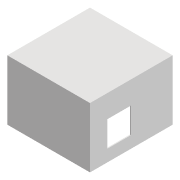
# Autodesk Inventor part: 玻璃罩
Saved by Autodesk Inventor 2021 (Build 250183000, 183)
## iProperties
Created: 2025-04-18
Part Number: 玻璃罩
Material: 常规
Document SubType Name: Modeling
Designer: 86155
Density: 1 g/cm^3
Appearance: 默认
Author: 86155
Autodesk Inventor part; units mm, degrees
ref_plane "YZ Plane" through (0, 0, 0) normal (1, 0, 0) x (0, 1, 0)
ref_plane "XZ Plane" through (0, 0, 0) normal (0, 1, 0) x (-1, 0, 0)
ref_plane "XY Plane" through (0, 0, 0) normal (0, 0, 1) x (1, 0, 0)
sketch "草图1" plane through (0, 0, 0) normal (0, 1, 0) x (-1, 0, 0)
  line L0 (410, 410) -> (-410, 410)
  line L1 (-410, 410) -> (-410, -410)
  line L2 (-410, -410) -> (410, -410)
  line L3 (410, -410) -> (410, 410)
  line L4 (410, 410) -> (-410, -410) construction
  line L5 (-410, 410) -> (410, -410) construction
  line L6 (420, 420) -> (-420, 420)
  line L7 (-420, 420) -> (-420, -420)
  line L8 (-420, -420) -> (420, -420)
  line L9 (420, -420) -> (420, 420)
  point P0 (0, 0)
  dimension "d0" = 820
  dimension "d1" = 820
  dimension "d2" = 10
  constraints: 20 end point, 4 parallel, 2 midpoint, 2 perpendicular, 1 horizontal, 3 other
  measures "d0" distance of L2.end L1.end
  measures "d1" distance of L1.end L0.end
  measures "d2" distance between parallel lines of L3 L9
extrude "拉伸1" add sketch "草图1" along normal blind 600
sketch "草图2" plane through (420, 0, -420) normal (0, 0, -1) x (-1, 0, 0)
  line L0 (49.0382, 250) -> (259.0382, 250)
  line L1 (259.0382, 250) -> (259.0382, 40)
  line L2 (259.0382, 40) -> (49.0382, 40)
  line L3 (49.0382, 40) -> (49.0382, 250)
  line L4 (0, 600) -> (840, 600) projected
  circle A0 centre (154.0382, 145) radius 50
  circle A1 centre (154.0382, 145) radius 40
  line L5 (154.0382, 145) -> (49.0382, 250)
  line L6 (154.0382, 145) -> (259.0382, 40)
  line L7 (49.0382, 40) -> (259.0382, 250)
  line L8 (63.1804, 40) -> (259.0382, 235.8579)
  line L9 (49.0382, 54.1421) -> (244.8961, 250)
  line L10 (49.0382, 235.8579) -> (146.9672, 137.9289)
  line L11 (146.9672, 137.9289) -> (244.8961, 40)
  line L12 (63.1804, 250) -> (161.1093, 152.0711)
  line L13 (161.1093, 152.0711) -> (259.0382, 54.1421)
  point P0 (420, 0)
  point P1 (188.4954, 165.3151)
  point P2 (133.7232, 110.5428)
  point P3 (174.3533, 179.4572)
  point P4 (119.581, 124.6849)
  point P5 (181.6082, 103.2879)
  point P6 (126.4683, 103.2879)
  point P7 (112.3261, 172.5699)
  point P8 (112.3261, 117.4301)
  point P9 (195.7503, 117.4301)
  point P10 (195.7503, 172.5699)
  point P11 (126.4683, 186.7121)
  point P12 (181.6082, 186.7121)
  dimension "d5" = 210
  dimension "d6" = 210
  dimension "d7" = 350
  dimension "d8" = 100
  dimension "d9" = 105
  dimension "d10" = 105
  dimension "d11" = 80
  dimension "d12" = 10
  dimension "d13" = 10
  dimension "d14" = 10
  dimension "d15" = 10
  constraints: 26 end point, 9 point on line, 4 parallel, 2 centre point, 1 coincident, 1 horizontal, 1 perpendicular
  measures "d5" distance of L1.end L2.end
  measures "d6" distance of L0.end L1.end
  measures "d7" distance between parallel lines of L4 L0
  measures "d8" diameter of A0
  measures "d9" distance from line of L2 A0.centre
  measures "d10" distance from line of L3 A0.centre
  measures "d11" diameter of A1
  measures "d12" distance between parallel lines of L7 L8
  measures "d13" distance between parallel lines of L7 L9
  measures "d14" distance between parallel lines of L6 L11
  measures "d15" distance between parallel lines of L6 L13
extrude "拉伸2" cut sketch "草图2" against normal blind 10 contours L0 L9 A0 L12 | L10 A0 L9 L3 | L5 L9 L10 A1 | A1 L12 L9 L5 | A1 L9 L12 | L10 L9 A1 | L1 L13 A0 L8 | L8 A0 L11 L2 | L8 L13 A1 L6 | L6 A1 L11 L8 | A1 L13 L8 | L8 L11 A1
sketch "草图3" plane through (0, 600, 0) normal (0, 1, 0) x (1, 0, 0)
  line L0 (-420, -420) -> (420, -420) projected
  line L1 (420, -420) -> (420, 420) projected
  line L2 (-420, -420) -> (420, -420)
  line L3 (420, -420) -> (420, 420)
  line L4 (420, 420) -> (-420, 420)
  line L5 (-420, 420) -> (-420, -420)
  point P0 (0, 0)
  constraints: 8 end point, 2 parallel, 1 horizontal, 1 perpendicular
extrude "拉伸3" add sketch "草图3" along normal blind 10
fillet "圆角1" radius 5 5 edges at (160.9618, 235.8579, -415) (175.1039, 250, -415) (238.3918, 186.7121, -415) (293.5317, 186.7121, -415) (356.8196, 250, -415)
fillet "圆角2" radius 5 11 edges at (224.2497, 172.5699, -415) (224.2497, 117.4301, -415) (356.8196, 40, -415) (370.9618, 235.8579, -415) (370.9618, 54.1421, -415) (160.9618, 54.1421, -415) (175.1039, 40, -415) (293.5317, 103.2879, -415) (238.3918, 103.2879, -415) (307.6739, 172.5699, -415) (307.6739, 117.4301, -415)
fillet "圆角3" radius 5 4 edges at (245.6467, 179.4572, -415) (231.5046, 165.3151, -415) (300.419, 124.6849, -415) (286.2768, 110.5428, -415)
sketch "草图4" plane through (420, 0, -420) normal (0, 0, -1) x (-1, 0, 0)
  line L0 (27.5194, 193.7371) -> (189.7881, 31.4684)
  line L1 (175.6459, 17.3263) -> (13.3773, 179.595)
  line L2 (57.5738, 227.3223) -> (109.5506, 175.3455) projected
  line L3 (27.5194, 193.7371) -> (13.3773, 179.595)
  line L4 (189.7881, 31.4684) -> (175.6459, 17.3263)
  line L5 (105.3011, 271.5188) -> (298.062, 78.758)
  line L6 (298.062, 78.758) -> (312.2041, 92.9001)
  line L7 (312.2041, 92.9001) -> (119.4433, 285.661)
  line L8 (119.4433, 285.661) -> (105.3011, 271.5188)
  line L9 (123.6927, 189.4876) -> (71.7159, 241.4645) projected
  point P0 (420, 0)
  dimension "d24" = 20
  dimension "d25" = 45
  dimension "d26" = 20
  dimension "d27" = 45
  constraints: 16 end point, 5 perpendicular, 1 point on line
  measures "d24" distance between parallel lines of L0 L1
  measures "d25" distance between parallel lines of L2 L0
  measures "d26" distance of L5.end L6.end
  measures "d27" distance between parallel lines of L9 L5
extrude "拉伸4" add sketch "草图4" against normal blind 10
sketch "草图5" plane through (420, 0, 420) normal (1, 0, 0) x (0, 0, -1)
  line L0 (175, 380) -> (415, 380)
  line L1 (415, 380) -> (415, 120)
  line L2 (415, 120) -> (175, 120)
  line L3 (175, 120) -> (175, 380)
  line L4 (0, 0) -> (0, 610) projected
  line L5 (0, 0) -> (840, 0) projected
  point P0 (420, 0)
  dimension "d30" = 260
  dimension "d31" = 240
  dimension "d32" = 175
  dimension "d33" = 120
  constraints: 8 end point, 2 parallel, 1 horizontal, 1 perpendicular
  measures "d30" distance between parallel lines of L2 L0
  measures "d31" distance between parallel lines of L1 L3
  measures "d32" distance between parallel lines of L4 L3
  measures "d33" distance between parallel lines of L5 L2
extrude "拉伸5" cut sketch "草图5" against normal blind 10
fillet "圆角4" radius 5 8 edges at (219.9998, 205.1041, -415) (264.8958, 250, -415) (205.8577, 190.9619, -415) (160.9618, 146.066, -415) (219.9998, 176.8198, -415) (160.9618, 117.7817, -415) (293.18, 250, -415) (234.142, 190.9619, -415)
fillet "圆角5" radius 5 4 edges at (370.9618, 172.2183, -415) (311.9237, 113.1802, -415) (297.7816, 99.0381, -415) (238.7435, 40, -415)
fillet "圆角6" radius 5 4 edges at (267.0278, 40, -415) (311.9237, 84.8959, -415) (326.0658, 99.0381, -415) (370.9618, 143.934, -415)
